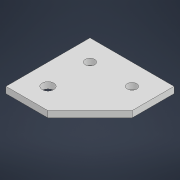
# Autodesk Inventor part: X-Axis End - Corner
Saved by Autodesk Inventor 2022 (Build 260153000, 153)
## iProperties
Created: 2023-06-22
Part Number: X-Axis End - Corner
Material: Generic
Document SubType Name: Modeling
Designer: Ryan Mitcham
Density: 1 g/cm^3
Appearance: Default
Author: Ryan Mitcham
Autodesk Inventor part; units mm, degrees
ref_plane "YZ Plane" through (0, 0, 0) normal (1, 0, 0) x (0, 1, 0)
ref_plane "XZ Plane" through (0, 0, 0) normal (0, 1, 0) x (-1, 0, 0)
ref_plane "XY Plane" through (0, 0, 0) normal (0, 0, 1) x (1, 0, 0)
sketch "Sketch1" plane through (0, 0, 0) normal (0, 1, 0) x (-1, 0, 0)
  line L0 (20, 20) -> (20, -20)
  line L1 (20, -20) -> (-20, -20)
  line L2 (-20, -20) -> (-20, 0)
  line L3 (20, 20) -> (0, 20)
  line L4 (0, 20) -> (-20, 0)
  point P0 (0, 0)
  point P1 (0, -20)
  point P2 (20, 0)
  dimension "d0" = 40
  dimension "d1" = 40
  dimension "d2" = 20
  dimension "d3" = 20
  constraints: 10 end point, 2 midpoint, 2 perpendicular, 1 horizontal, 1 horizontal alignment, 1 vertical, 1 vertical alignment
  measures "d0" distance of L0.start L0.end
  measures "d1" distance of L0.end L1.end
  measures "d2" distance of L1.end L2.end
  measures "d3" distance of L0.start L3.end
extrude "Extrusion1" add sketch "Sketch1" along normal blind 3
sketch "Sketch2" plane through (0, 3, 0) normal (0, 1, 0) x (1, 0, 0)
  line L0 (-20, 20) -> (-20, -20) projected
  line L1 (20, 0) -> (20, 20) projected
  line L2 (20, 20) -> (-20, 20) projected
  point P0 (0, 0)
  point P1 (-10, 10)
  point P2 (10, 10)
  dimension "d6" = 10
  dimension "d7" = 10
  dimension "d8" = 10
  constraints: 1 horizontal alignment
  measures "d6" distance from line of L0 point (-10, 10)
  measures "d7" distance from line of L1 point (10, 10)
  measures "d8" distance from line of L2 point (-10, 10)
hole "Hole1" at (-10, 3, -10) at (10, 3, -10) direction (0, -1, 0) diameter 4.5 end through all
sketch "Sketch3" plane through (0, 3, 0) normal (0, 1, 0) x (1, 0, 0)
  line L0 (-20, -20) -> (0, -20) projected
  line L1 (-20, 20) -> (-20, -20) projected
  point P0 (0, 0)
  point P1 (-10, -10)
  dimension "d16" = 10
  dimension "d17" = 10
  measures "d16" distance from line of L0 point (-10, -10)
  measures "d17" distance from line of L1 point (-10, -10)
hole "Hole2" at (-10, 3, 10) direction (0, -1, 0) diameter 5.5 end through all
equation "\"d1\" = d0"
body "Solid1"
